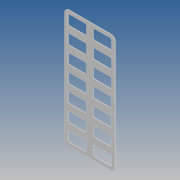
# Autodesk Inventor part: front_Box
Saved by Autodesk Inventor 2020 (Build 240168000, 168)
## iProperties
Created: 2020-07-14
Part Number: front_Box
Material: Générique
Document SubType Name: Modeling
Designer: carmine.arcudi
Density: 1 g/cm^3
Appearance: Par défaut
Author: carmine.arcudi
Autodesk Inventor part; units mm, degrees
ref_plane "YZ Plane" through (0, 0, 0) normal (1, 0, 0) x (0, 1, 0)
ref_plane "XZ Plane" through (0, 0, 0) normal (0, 1, 0) x (-1, 0, 0)
ref_plane "XY Plane" through (0, 0, 0) normal (0, 0, 1) x (1, 0, 0)
sketch "Esquisse1" plane through (0, 0, 0) normal (0, 0, 1) x (1, 0, 0)
  line L0 (-120, 336) -> (120, 336)
  line L1 (144, 312) -> (144, -312)
  line L2 (120, -336) -> (-120, -336)
  line L3 (-144, -312) -> (-144, 312)
  arc A0 (-120, 336) -> (-144, 312) centre (-120, 312) ccw
  arc A1 (144, 312) -> (120, 336) centre (120, 312) ccw
  arc A2 (120, -336) -> (144, -312) centre (120, -312) ccw
  arc A3 (-144, -312) -> (-120, -336) centre (-120, -312) ccw
  line L4 (24, -259) -> (120, -259)
  line L5 (125, -264) -> (125, -312)
  line L6 (120, -317) -> (24, -317)
  line L7 (19, -312) -> (19, -264)
  line L8 (24, -259) -> (19, -264)
  line L9 (120, -259) -> (125, -264)
  line L10 (125, -312) -> (120, -317)
  line L11 (24, -317) -> (19, -312)
  line L12 (24, -163) -> (19, -168)
  line L13 (24, -163) -> (120, -163)
  line L14 (120, -163) -> (125, -168)
  line L15 (19, -216) -> (19, -168)
  line L16 (24, -221) -> (19, -216)
  line L17 (120, -221) -> (24, -221)
  line L18 (125, -168) -> (125, -216)
  line L19 (125, -216) -> (120, -221)
  line L20 (24, -67) -> (19, -72)
  line L21 (24, -67) -> (120, -67)
  line L22 (120, -67) -> (125, -72)
  line L23 (19, -120) -> (19, -72)
  line L24 (24, -125) -> (19, -120)
  line L25 (120, -125) -> (24, -125)
  line L26 (125, -72) -> (125, -120)
  line L27 (125, -120) -> (120, -125)
  line L28 (24, 29) -> (19, 24)
  line L29 (24, 29) -> (120, 29)
  line L30 (120, 29) -> (125, 24)
  line L31 (19, -24) -> (19, 24)
  line L32 (24, -29) -> (19, -24)
  line L33 (120, -29) -> (24, -29)
  line L34 (125, 24) -> (125, -24)
  line L35 (125, -24) -> (120, -29)
  line L36 (24, 125) -> (19, 120)
  line L37 (24, 125) -> (120, 125)
  line L38 (120, 125) -> (125, 120)
  line L39 (19, 72) -> (19, 120)
  line L40 (24, 67) -> (19, 72)
  line L41 (120, 67) -> (24, 67)
  line L42 (125, 120) -> (125, 72)
  line L43 (125, 72) -> (120, 67)
  line L44 (24, 221) -> (19, 216)
  line L45 (24, 221) -> (120, 221)
  line L46 (120, 221) -> (125, 216)
  line L47 (19, 168) -> (19, 216)
  line L48 (24, 163) -> (19, 168)
  line L49 (120, 163) -> (24, 163)
  line L50 (125, 216) -> (125, 168)
  line L51 (125, 168) -> (120, 163)
  line L52 (24, 317) -> (19, 312)
  line L53 (24, 317) -> (120, 317)
  line L54 (120, 317) -> (125, 312)
  line L55 (19, 264) -> (19, 312)
  line L56 (24, 259) -> (19, 264)
  line L57 (120, 259) -> (24, 259)
  line L58 (125, 312) -> (125, 264)
  line L59 (125, 264) -> (120, 259)
  line L60 (-120, -259) -> (-125, -264)
  line L61 (-120, -259) -> (-24, -259)
  line L62 (-24, -259) -> (-19, -264)
  line L63 (-125, -312) -> (-125, -264)
  line L64 (-120, -317) -> (-125, -312)
  line L65 (-24, -317) -> (-120, -317)
  line L66 (-19, -264) -> (-19, -312)
  line L67 (-19, -312) -> (-24, -317)
  line L68 (-120, -163) -> (-125, -168)
  line L69 (-120, -163) -> (-24, -163)
  line L70 (-24, -163) -> (-19, -168)
  line L71 (-125, -216) -> (-125, -168)
  line L72 (-120, -221) -> (-125, -216)
  line L73 (-24, -221) -> (-120, -221)
  line L74 (-19, -168) -> (-19, -216)
  line L75 (-19, -216) -> (-24, -221)
  line L76 (-120, -67) -> (-125, -72)
  line L77 (-120, -67) -> (-24, -67)
  line L78 (-24, -67) -> (-19, -72)
  line L79 (-125, -120) -> (-125, -72)
  line L80 (-120, -125) -> (-125, -120)
  line L81 (-24, -125) -> (-120, -125)
  line L82 (-19, -72) -> (-19, -120)
  line L83 (-19, -120) -> (-24, -125)
  line L84 (-120, 29) -> (-125, 24)
  line L85 (-120, 29) -> (-24, 29)
  line L86 (-24, 29) -> (-19, 24)
  line L87 (-125, -24) -> (-125, 24)
  line L88 (-120, -29) -> (-125, -24)
  line L89 (-24, -29) -> (-120, -29)
  line L90 (-19, 24) -> (-19, -24)
  line L91 (-19, -24) -> (-24, -29)
  line L92 (-120, 125) -> (-125, 120)
  line L93 (-120, 125) -> (-24, 125)
  line L94 (-24, 125) -> (-19, 120)
  line L95 (-125, 72) -> (-125, 120)
  line L96 (-120, 67) -> (-125, 72)
  line L97 (-24, 67) -> (-120, 67)
  line L98 (-19, 120) -> (-19, 72)
  line L99 (-19, 72) -> (-24, 67)
  line L100 (-120, 221) -> (-125, 216)
  line L101 (-120, 221) -> (-24, 221)
  line L102 (-24, 221) -> (-19, 216)
  line L103 (-125, 168) -> (-125, 216)
  line L104 (-120, 163) -> (-125, 168)
  line L105 (-24, 163) -> (-120, 163)
  line L106 (-19, 216) -> (-19, 168)
  line L107 (-19, 168) -> (-24, 163)
  line L108 (-120, 317) -> (-125, 312)
  line L109 (-120, 317) -> (-24, 317)
  line L110 (-24, 317) -> (-19, 312)
  line L111 (-125, 264) -> (-125, 312)
  line L112 (-120, 259) -> (-125, 264)
  line L113 (-24, 259) -> (-120, 259)
  line L114 (-19, 312) -> (-19, 264)
  line L115 (-19, 264) -> (-24, 259)
  circle A4 centre (130, -322) radius 1.25
  circle A5 centre (130, 322) radius 1.25
  circle A6 centre (0, -322) radius 1.25
  circle A7 centre (0, 322) radius 1.25
  circle A8 centre (-130, -322) radius 1.25
  circle A9 centre (-130, 322) radius 1.25
  circle A10 centre (130, -240) radius 1.25
  circle A11 centre (130, -144) radius 1.25
  circle A12 centre (130, -48) radius 1.25
  circle A13 centre (130, 48) radius 1.25
  circle A14 centre (130, 144) radius 1.25
  circle A15 centre (130, 240) radius 1.25
  circle A16 centre (0, -240) radius 1.25
  circle A17 centre (0, -144) radius 1.25
  circle A18 centre (0, -48) radius 1.25
  circle A19 centre (0, 48) radius 1.25
  circle A20 centre (0, 144) radius 1.25
  circle A21 centre (0, 240) radius 1.25
  circle A22 centre (-130, -240) radius 1.25
  circle A23 centre (-130, -144) radius 1.25
  circle A24 centre (-130, -48) radius 1.25
  circle A25 centre (-130, 48) radius 1.25
  circle A26 centre (-130, 144) radius 1.25
  circle A27 centre (-130, 240) radius 1.25
  point P0 (0, 0)
  point P1 (-144, 336)
  point P2 (144, 336)
  point P3 (-144, -336)
  point P4 (19, -259)
  point P5 (125, -317)
  point P6 (125, -259)
  point P7 (19, -317)
  point P8 (19, -163)
  point P9 (125, -163)
  point P10 (19, -221)
  point P11 (125, -221)
  point P12 (120, -216)
  point P13 (19, -67)
  point P14 (125, -67)
  point P15 (19, -125)
  point P16 (125, -125)
  point P17 (120, -120)
  point P18 (19, 29)
  point P19 (125, 29)
  point P20 (19, -29)
  point P21 (125, -29)
  point P22 (120, -24)
  point P23 (19, 125)
  point P24 (125, 125)
  point P25 (19, 67)
  point P26 (125, 67)
  point P27 (120, 72)
  point P28 (19, 221)
  point P29 (125, 221)
  point P30 (19, 163)
  point P31 (125, 163)
  point P32 (120, 168)
  point P33 (19, 317)
  point P34 (125, 317)
  point P35 (19, 259)
  point P36 (125, 259)
  point P37 (120, 264)
  point P38 (-125, -259)
  point P39 (-19, -259)
  point P40 (-125, -317)
  point P41 (-19, -317)
  point P42 (-24, -312)
  point P43 (-125, -163)
  point P44 (-19, -163)
  point P45 (-125, -221)
  point P46 (-19, -221)
  point P47 (-24, -216)
  point P48 (-125, -67)
  point P49 (-19, -67)
  point P50 (-125, -125)
  point P51 (-19, -125)
  point P52 (-24, -120)
  point P53 (-125, 29)
  point P54 (-19, 29)
  point P55 (-125, -29)
  point P56 (-19, -29)
  point P57 (-24, -24)
  point P58 (-125, 125)
  point P59 (-19, 125)
  point P60 (-125, 67)
  point P61 (-19, 67)
  point P62 (-24, 72)
  point P63 (-125, 221)
  point P64 (-19, 221)
  point P65 (-125, 163)
  point P66 (-19, 163)
  point P67 (-24, 168)
  point P68 (-125, 317)
  point P69 (-19, 317)
  point P70 (-125, 259)
  point P71 (-19, 259)
  point P72 (-24, 264)
  dimension "d0" = 672
  dimension "d1" = 288
  dimension "d2" = 144
  dimension "d3" = 336
  dimension "d4" = 24
  dimension "d5" = 106
  dimension "d6" = 58
  dimension "d7" = 19
  dimension "d8" = 19
  dimension "d9" = 5
  dimension "d10" = 5
  dimension "d11" = 5
  dimension "d12" = 5
  dimension "d13" = 5
  dimension "d14" = 5
  dimension "d15" = 5
  dimension "d16" = 5
  dimension "d19" = 96
  dimension "d22" = 144
  dimension "d25" = 2.5
  dimension "d26" = 14
  dimension "d27" = 14
  dimension "d30" = 644
  dimension "d33" = 130
  dimension "d36" = 2.5
  dimension "d37" = 14
  dimension "d38" = 96
  dimension "d41" = 96
  dimension "d44" = 130
  constraints: 232 end point, 118 point on line, 28 centre point, 8 point on circle, 8 tangent, 5 horizontal, 4 parallel, 3 equal radius, 3 vertical, 2 perpendicular, 317 other
  measures "d0" distance of point (-144, -336) point (-144, 336)
  measures "d1" distance of point (-144, 336) point (144, 336)
  measures "d2" distance from line of L3 point (0, 0)
  measures "d3" distance from line of point (0, 0) L0
  measures "d4" radius of A0
  measures "d5" distance of point (19, -259) point (125, -259)
  measures "d6" distance of point (19, -317) point (19, -259)
  measures "d7" distance between parallel lines of L6 L2
  measures "d8" distance between parallel lines of L1 L5
  measures "d9" distance of L4.start point (19, -259)
  measures "d10" distance of L7.end point (19, -259)
  measures "d11" distance of L4.end point (125, -259)
  measures "d12" distance of L5.start point (125, -259)
  measures "d13" distance of L5.end point (125, -317)
  measures "d14" distance of L6.start point (125, -317)
  measures "d15" distance of L6.end point (19, -317)
  measures "d16" distance of L7.start point (19, -317)
  measures "d19" distance of point (19, -259) point (19, -163)
  measures "d22" distance of point (19, -259) point (-125, -259)
  measures "d25" diameter of A4
  measures "d26" distance from line of L2 A4.centre
  measures "d27" distance from line of L1 A4.centre
  measures "d30" distance of A4.centre A5.centre
  measures "d33" distance of A4.centre A6.centre
  measures "d36" diameter of A10
  measures "d37" distance from line of L1 A10.centre
  measures "d38" distance from line of A10.centre L2
  measures "d41" distance of A10.centre A11.centre
  measures "d44" distance of A10.centre A16.centre
extrude "Extrusion1" add sketch "Esquisse1" along normal blind 3
equation "\"d2\" = 0.5 * d1"
equation "\"d3\" = 0.5 * d0"
equation "\"d10\" = d9"
equation "\"d11\" = d9"
equation "\"d12\" = d11"
equation "\"d13\" = d9"
equation "\"d14\" = d13"
equation "\"d15\" = d9"
equation "\"d16\" = d15"
